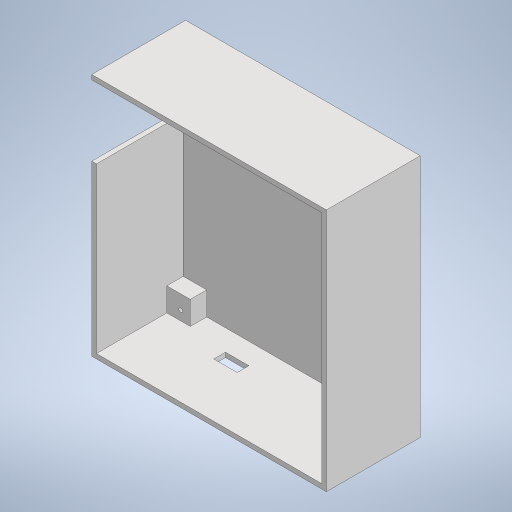
# Autodesk Inventor part: e_box
Saved by Autodesk Inventor 2024.1 (Build 281209000, 209)
## iProperties
Created: 2023-10-07
Part Number: e_box
Material: Generic
Document SubType Name: Modeling
Designer: l1534
Density: 1 g/cm^3
Appearance: Default
Author: l1534
Autodesk Inventor part; units mm, degrees
ref_plane "YZ Plane" through (0, 0, 0) normal (1, 0, 0) x (0, 1, 0)
ref_plane "XZ Plane" through (0, 0, 0) normal (0, 1, 0) x (-1, 0, 0)
ref_plane "XY Plane" through (0, 0, 0) normal (0, 0, 1) x (1, 0, 0)
sketch "Sketch1" plane through (0, 0, 0) normal (0, 0, 1) x (1, 0, 0)
  line L0 (-65.4164, 28.1839) -> (34.5836, 28.1839)
  line L1 (34.5836, 28.1839) -> (34.5836, -75.8161)
  line L2 (34.5836, -75.8161) -> (-65.4164, -75.8161)
  line L3 (-65.4164, -75.8161) -> (-65.4164, 28.1839)
  point P0 (0, 0)
  dimension "d0" = 100
  dimension "d1" = 104
  constraints: 8 end point, 2 parallel, 1 horizontal, 1 perpendicular
  measures "d0" distance of L0.start L0.end
  measures "d1" distance of L0.end L1.end
extrude "Extrusion1" add sketch "Sketch1" along normal blind 40
sketch "Sketch2" plane through (0, 0, 40) normal (0, 0, 1) x (1, 0, 0)
  line L0 (-63.4164, 26.1839) -> (32.5836, 26.1839)
  line L1 (32.5836, 26.1839) -> (32.5836, -73.8161)
  line L2 (32.5836, -73.8161) -> (-63.4164, -73.8161)
  line L3 (-63.4164, -73.8161) -> (-63.4164, 26.1839)
  line L4 (34.5836, 28.1839) -> (-65.4164, 28.1839) projected
  line L5 (34.5836, -75.8161) -> (34.5836, 28.1839) projected
  line L6 (-65.4164, 28.1839) -> (-65.4164, -75.8161) projected
  line L7 (-65.4164, -75.8161) -> (34.5836, -75.8161) projected
  point P0 (0, 0)
  dimension "d4" = 2
  dimension "d5" = 2
  dimension "d6" = 2
  dimension "d7" = 2
  constraints: 8 end point, 2 parallel, 1 horizontal, 1 perpendicular
  measures "d4" distance between parallel lines of L4 L0
  measures "d5" distance between parallel lines of L5 L1
  measures "d6" distance between parallel lines of L6 L3
  measures "d7" distance between parallel lines of L7 L2
extrude "Extrusion2" cut sketch "Sketch2" against normal blind 37 contours L0 L1 L2 L3
sketch "Sketch3" plane through (0, 0, 3) normal (0, 0, 1) x (1, 0, 0)
  line L0 (-63.4164, 26.1839) -> (32.5836, 26.1839) projected
  line L1 (-63.4164, 26.1839) -> (-53.4164, 26.1839)
  line L2 (-53.4164, 26.1839) -> (-53.4164, 16.1839)
  line L3 (-53.4164, 16.1839) -> (-63.4164, 16.1839)
  line L4 (-63.4164, 16.1839) -> (-63.4164, 26.1839)
  line L5 (32.5836, 26.1839) -> (22.5836, 26.1839)
  line L6 (22.5836, 26.1839) -> (22.5836, 16.1839)
  line L7 (22.5836, 16.1839) -> (32.5836, 16.1839)
  line L8 (32.5836, 16.1839) -> (32.5836, 26.1839)
  line L9 (32.5836, -73.8161) -> (-63.4164, -73.8161) projected
  line L10 (-63.4164, -73.8161) -> (-53.4164, -73.8161)
  line L11 (-53.4164, -73.8161) -> (-53.4164, -63.8161)
  line L12 (-53.4164, -63.8161) -> (-63.4164, -63.8161)
  line L13 (-63.4164, -63.8161) -> (-63.4164, -73.8161)
  line L14 (32.5836, -73.8161) -> (22.5836, -73.8161)
  line L15 (22.5836, -73.8161) -> (22.5836, -63.8161)
  line L16 (22.5836, -63.8161) -> (32.5836, -63.8161)
  line L17 (32.5836, -63.8161) -> (32.5836, -73.8161)
  point P0 (0, 0)
  dimension "d10" = 10
  dimension "d11" = 10
  dimension "d12" = 10
  dimension "d13" = 10
  dimension "d14" = 10
  dimension "d15" = 10
  dimension "d16" = 10
  dimension "d17" = 10
  constraints: 32 end point, 8 parallel, 4 horizontal, 4 perpendicular
  measures "d10" distance of L2.end L3.end
  measures "d11" distance of L1.end L2.end
  measures "d12" distance of L5.end L6.end
  measures "d13" distance of L6.end L7.end
  measures "d14" distance of L11.end L12.end
  measures "d15" distance of L10.end L11.end
  measures "d16" distance of L14.end L15.end
  measures "d17" distance of L15.end L16.end
extrude "Extrusion3" add sketch "Sketch3" along normal blind 7
sketch "Sketch4" plane through (0, 0, 40) normal (0, 0, 1) x (1, 0, 0)
  line L0 (-65.4164, 28.1839) -> (-65.4164, -75.8161) projected
  line L1 (-63.4164, 26.1839) -> (-65.4164, 26.1839)
  line L2 (-65.4164, 26.1839) -> (-65.4164, -3.8161)
  line L3 (-65.4164, -3.8161) -> (-63.4164, -3.8161)
  line L4 (-63.4164, -3.8161) -> (-63.4164, 26.1839)
  point P0 (0, 0)
  dimension "d20" = 30
  constraints: 8 end point, 2 parallel, 1 horizontal, 1 perpendicular, 1 point on line
  measures "d20" distance between parallel lines of L3 L1
extrude "Extrusion4" cut sketch "Sketch4" against normal up to surface (30 mm away)
sketch "Sketch5" plane through (0, 0, 10) normal (0, 0, 1) x (1, 0, 0)
  line L0 (-53.4164, 16.1839) -> (-63.4164, 16.1839) projected
  line L1 (-65.4164, 28.1839) -> (-65.4164, -75.8161) projected
  line L2 (-63.4164, 16.1839) -> (-65.4164, 16.1839)
  line L3 (-65.4164, 16.1839) -> (-65.4164, -3.8161)
  line L4 (-65.4164, -3.8161) -> (-63.4164, -3.8161)
  line L5 (-63.4164, -3.8161) -> (-63.4164, 16.1839)
  point P0 (0, 0)
  dimension "d23" = 20
  constraints: 8 end point, 2 parallel, 1 horizontal, 1 perpendicular, 1 point on line
  measures "d23" distance of L4.end L0.end
extrude "Extrusion5" cut sketch "Sketch5" against normal up to surface (7 mm away)
sketch "Sketch6" plane through (0, 0, 10) normal (0, 0, 1) x (1, 0, 0)
  circle A0 centre (-57.5414, 22.1839) radius 0.8
  circle A1 centre (26.7086, 22.1839) radius 0.8
  circle A2 centre (26.7086, -69.8161) radius 0.8
  circle A3 centre (-57.5414, -69.8161) radius 0.8
  line L0 (32.5836, -73.8161) -> (-63.4164, -73.8161) projected
  line L1 (32.5836, 26.1839) -> (32.5836, -73.8161) projected
  line L2 (-63.4164, -73.8161) -> (-63.4164, -3.8161) projected
  line L3 (-65.4164, 26.1839) -> (32.5836, 26.1839) projected
  point P0 (0, 0)
  dimension "d26" = 1.6
  dimension "d27" = 1.6
  dimension "d28" = 1.6
  dimension "d29" = 1.6
  dimension "d30" = 4
  dimension "d31" = 5.875
  dimension "d32" = 4
  dimension "d33" = 5.875
  dimension "d34" = 5.875
  dimension "d35" = 5.875
  dimension "d36" = 4
  dimension "d37" = 4
  constraints: 4 centre point
  measures "d26" diameter of A0
  measures "d27" diameter of A1
  measures "d28" diameter of A2
  measures "d29" diameter of A3
  measures "d30" distance from line of L0 A2.centre
  measures "d31" distance from line of L1 A2.centre
  measures "d32" distance from line of L0 A3.centre
  measures "d33" distance from line of L2 A3.centre
  measures "d34" distance from line of L1 A1.centre
  measures "d35" distance from line of L2 A0.centre
  measures "d36" distance from line of L3 A0.centre
  measures "d37" distance from line of L3 A1.centre
extrude "Extrusion6" cut sketch "Sketch6" against normal through all
sketch "Sketch7" plane through (-63.4164, -73.8161, 40) normal (0, 1, 0) x (1, 0, 0)
  line L0 (27, 23) -> (37, 23)
  line L1 (37, 23) -> (37, 28)
  line L2 (37, 28) -> (27, 28)
  line L3 (27, 28) -> (27, 23)
  line L4 (0, 0) -> (0, 30) projected
  line L5 (86, 37) -> (10, 37) projected
  point P0 (63.4164, 40)
  dimension "d40" = 10
  dimension "d41" = 5
  dimension "d42" = 27
  dimension "d43" = 9
  constraints: 8 end point, 2 parallel, 1 horizontal, 1 perpendicular
  measures "d40" distance of L0.start L0.end
  measures "d41" distance of L2.end L0.start
  measures "d42" distance between parallel lines of L4 L3
  measures "d43" distance between parallel lines of L5 L2
extrude "Extrusion7" cut sketch "Sketch7" against normal through all
body "Solid1"
